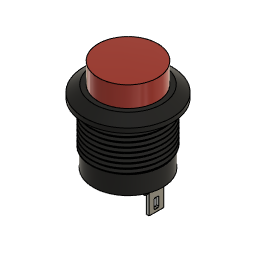
PushButtonRed v9 (Autodesk Fusion 360 design; units mm, degrees)
Autodesk Fusion 360 part; units mm, degrees
sketch "ButtonShell" plane through (0, 0, 0) normal (0, 1, 0) x (1, 0, 0) in component "ButtonBody"
  line L0 (0, 0) -> (9.65, 0)
  line L1 (9.65, 0) -> (9.65, -1)
  line L2 (0, -2.5) -> (9.65, -2.5) construction
  line L3 (0, -2.5) -> (7.5, -2.5)
  line L4 (7.5, -2.5) -> (9.65, -1)
  line L5 (0, -2.5) -> (0, 0)
  dimension "d17" = 9.65
  dimension "d19" = 1
  dimension "d20" = 2.5
  dimension "d21" = 7.5
  constraint coincident L0.start L5.end
  constraint horizontal L0
  constraint perpendicular L0 L1
  constraint parallel L2 L3
  constraint perpendicular L0 L5
  measures "d17" distance of L0.start L0.end
  measures "d19" distance of L0.end L1.end
  measures "d21" distance of L2.start L3.end
revolve "Revolve1" add sketch "ButtonShell" angle 360 about axis through (0, 0, 2.5) along (0, 0, -1) makes body 1 in component "ButtonBody"
sketch "ButtonBody" plane through (0, 0, 0) normal (0, 0, -1) x (1, 0, 0) in component "ButtonBody"
  circle A0 centre (0, 0) radius 9.65
  circle A1 centre (0, 0) radius 7.6
  circle A2 centre (0, 0) radius 8
  dimension "d23" = 15.2
  dimension "d24" = 16
  constraint coincident A0.centre A1.centre
  measures "d23" diameter of A1
  measures "d24" diameter of A2
extrude "Extrude1" add sketch "ButtonBody" along normal blind 13.3 contours A1 bodies 1 in component "ButtonBody"
extrude "Extrude2" add sketch "ButtonBody" along normal blind 9.3 contours A2 bodies 1 in component "ButtonBody"
thread "Thread1" "ISO Metric profile 16.0 M16x1 6g" major diameter 15.884 minor diameter 14.741 pitch 1 angle 60 modelled right hand crest width 0.1429 on face at (7.9901, 0.3988, -6.2) crest through (7.942, 0, 0.25) on bodies 1 in component "ButtonBody"
sketch "ButtonBase" plane through (0, 0, 2.5) normal (0, 0, 1) x (-1, 0, 0) in component "Button"
  circle A0 centre (0, 0) radius 7.5
  circle A1 centre (0, 0) radius 6.5
  dimension "d29" = 13
  constraint concentric A0 A1
  measures "d29" diameter of A1
extrude "Extrude1'" add sketch "ButtonBase" along normal blind 4.5 separate body contours A1 makes body 2 in component "Button"
sketch "ConnectorBase" plane through (0, 0, 0) normal (0, 1, 0) x (1, 0, 0) in component "Connector"
  line L0 (0, 0) -> (5, 0)
  line L1 (5, 0) -> (5, -1)
  line L2 (5, -1) -> (4.1, -1)
  line L3 (4.1, -1) -> (4.1, -5.3)
  line L4 (4.1, -5.3) -> (0.9, -5.3)
  line L5 (0.9, -5.3) -> (0.9, -1)
  line L6 (0.9, -1) -> (0, -1)
  line L7 (0, -1) -> (0, 0)
  line L8 (4.1, -3.6) -> (0.9, -3.6) construction
  line L9 (2.5, -3.6) -> (2.5, -2.5) construction
  line L10 (2.5, -3.6) -> (2.5, -4.7) construction
  line L11 (3, -3.6) -> (3, -4.5) construction
  line L12 (3, -3.6) -> (3, -2.7) construction
  line L13 (2, -3.6) -> (2, -4.5) construction
  line L14 (2, -3.6) -> (2, -2.7) construction
  line L15 (2.2, -2.5) -> (2.8, -2.5)
  line L16 (3, -2.5) -> (3, -4.7)
  line L17 (2.8, -4.7) -> (2.2, -4.7)
  line L18 (2, -4.7) -> (2, -2.5)
  arc A0 (2.8, -4.7) -> (3, -4.5) centre (2.8, -4.5) ccw
  arc A1 (3, -2.7) -> (2.8, -2.5) centre (2.8, -2.7) ccw
  arc A2 (2.2, -2.5) -> (2, -2.7) centre (2.2, -2.7) ccw
  arc A3 (2, -4.5) -> (2.2, -4.7) centre (2.2, -4.5) ccw
  dimension "d32" = 5
  dimension "d35" = 1
  dimension "d36" = 0.9
  dimension "d37" = 4.3
  dimension "d39" = 3.2
  dimension "d40" = 4.3
  dimension "d41" = 0.9
  dimension "d42" = 1.7
  dimension "d43" = 1.1
  dimension "d44" = 1.1
  dimension "d47" = 0.2
  constraint coincident L0.start L7.end
  constraint horizontal L0
  constraint perpendicular L0 L1
  constraint perpendicular L1 L2
  constraint perpendicular L2 L3
  constraint perpendicular L3 L4
  constraint perpendicular L4 L5
  constraint perpendicular L5 L6
  constraint midpoint L8 L9.start
  constraint perpendicular L8 L9
  constraint perpendicular L8 L10
  constraint horizontal L15
  constraint vertical L16
  constraint horizontal L17
  constraint vertical L18
  constraint parallel L10 L11
  constraint parallel L9 L12
  constraint coincident L16.end L17
  constraint coincident L16.end L11
  constraint tangent L17 A0
  constraint tangent L11 A0
  constraint coincident L16.start L15
  constraint tangent L12 A1
  constraint tangent L15 A1
  constraint equal A0 A1
  constraint parallel L10 L13
  constraint parallel L9 L14
  constraint coincident L18.end L14
  constraint coincident L18.end L15
  constraint tangent L14 A2
  constraint tangent L15 A2
  constraint equal A0 A2
  constraint coincident L18.start L17
  constraint tangent L17 A3
  constraint tangent L13 A3
  constraint equal A0 A3
  measures "d32" distance of L0.start L0.end
  measures "d35" distance of L0.end L1.end
  measures "d36" distance of L1.end L2.end
  measures "d37" distance of L2.end L3.end
  measures "d39" distance of L3.end L4.end
  measures "d40" distance of L4.end L5.end
  measures "d41" distance of L5.end L6.end
  measures "d43" distance of L9.start L9.end
  measures "d44" distance of L9.start L10.end
  measures "d47" radius of A0
extrude "Extrude1''" add sketch "ConnectorBase" along normal blind 0.6 separate body makes body 3 in component "Connector"
sketch "ConnectorsPosition" plane through (0, 0, -13.3) normal (0, 0, -1) x (1, 0, 0) in component "ButtonBody"
  circle A0 centre (0, 0) radius 7.6
  circle A1 centre (0, 0) radius 5.95 construction
  line L0 (0, 0) -> (-5.95, 0) construction
  line L1 (0, 0) -> (5.95, 0) construction
  dimension "d50" = 11.9
  constraint concentric A0 A1
  constraint coincident A0.centre A1.centre
  constraint coincident A1 L0.end
  constraint horizontal L0
  constraint coincident A1 L1.end
  constraint parallel L0 L1
  measures "d50" diameter of A1
sketch "Sketch1" plane through (0, 0, 0) normal (0, 0, 1) x (1, 0, 0) in component "Nut"
  line L0 (-9.5, -5.4848) -> (0, -10.9697)
  line L1 (0, -10.9697) -> (9.5, -5.4848)
  line L2 (9.5, -5.4848) -> (9.5, 5.4848)
  line L3 (9.5, 5.4848) -> (0, 10.9697)
  line L4 (0, 10.9697) -> (-9.5, 5.4848)
  line L5 (-9.5, 5.4848) -> (-9.5, -5.4848)
  circle A0 centre (0, 0) radius 8
  dimension "d64" = 9.5
  dimension "d65" = 16
  constraint coincident A0.centre origin
  measures "d64" distance of A0.centre L5
  measures "d65" diameter of A0
extrude "Extrude1'''" add sketch "Sketch1" along normal blind 2.5 separate body makes body 4 in component "Nut"
thread "Thread1'" "ISO Metric profile 16.0 M16x1 6H" major diameter 16.1522 minor diameter 15.0355 pitch 1 angle 60 modelled right hand crest width 0.2719 on face at (7.9901, -0.3988, 1.6667) crest through (7.5178, 0, 0.25) on bodies 4 in component "Nut"
component "ButtonBody" placed x (1, 0, 0) y (0, 1, 0) z (0, 0, 1) at (0, 0, 0)
component "Button" placed x (1, 0, 0) y (0, 1, 0) z (0, 0, 1) at (0, 0, 0)
component "Connector" placed x (0, -1, 0) y (-1, 0, 0) z (0, 0, -1) at (-5.65, 2.5, -13.3)
component "Connector" placed x (0, -1, 0) y (-1, 0, 0) z (0, 0, -1) at (6.25, 2.5, -13.3)
component "Nut" placed x (1, 0, 0) y (0, 1, 0) z (0, 0, 1) at (0, 0, -2.5)
equation "ButtonShellDiameter = 19.3 mm"
equation "ButtonDiameter = 13 mm"
equation "ButtonShellHeight = 2.5 mm"
equation "ButtonHeight = 4.5 mm"
equation "ButtonBodyDiameter = 15.2 mm"
equation "ButtonScrewDiameter = 16 mm"
equation "ButtonBodyHeight = 13.3 mm"
equation "ButtonScrewHeight = 9.3 mm"
equation "ButtonScrewSpacing = 1 mm"
equation "ConnectorsOffset = 3 mm"
equation "ConnectorWidth = 0.6 mm"
equation "ConnectorBaseLenght = 5 mm"
equation "ConnectorTipLenght = 3.2 mm"
equation "ConnectorHolePositionFromTop = 1.7 mm"
equation "ConnectorHoleHeight = 2.2 mm"
equation "ConnectorHoleWidth = 1 mm"
equation "d17 = ButtonShellDiameter / 2"
equation "ButtonShellBaseHeight = 1 mm"
equation "d19 = ButtonShellBaseHeight"
equation "d20 = ButtonShellHeight"
equation "d21 = 6.50 mm + 1 mm"
equation "d23 = ButtonBodyDiameter"
equation "d24 = ButtonScrewDiameter"
equation "d25 = ButtonBodyHeight"
equation "d27 = ButtonScrewHeight"
equation "d29 = ButtonDiameter"
equation "d30 = ButtonHeight"
equation "d32 = ConnectorBaseLenght"
equation "ConnectorHeight = 5.3 mm"
equation "ConnectorBaseHeight = 1 mm"
equation "d35 = ConnectorBaseHeight"
equation "d36 = ConnectorBaseLenght / 2 - ConnectorTipLenght / 2"
equation "d37 = ConnectorHeight - ConnectorBaseHeight"
equation "d39 = ConnectorTipLenght"
equation "d40 = d37"
equation "d41 = d36"
equation "d42 = ConnectorHolePositionFromTop"
equation "d43 = ConnectorHoleHeight / 2"
equation "d44 = d43"
equation "d48 = ConnectorWidth"
equation "d50 = ButtonBodyDiameter - ( ConnectorsOffset + ConnectorWidth / 2 )"
equation "NutDiameter = 19 mm"
equation "d64 = NutDiameter / 2"
equation "d65 = ButtonScrewDiameter"
equation "NutHeight = 2.5 mm"
equation "d67 = NutHeight"
